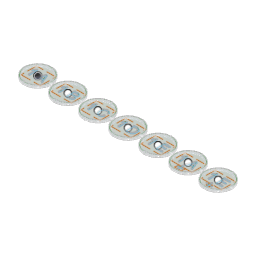
_Marker Chip 1A.5286f14f-15ed-4947-bf56-e78f0308ec14 (Autodesk Fusion 360 design; units mm, degrees)
Autodesk Fusion 360 part; units mm, degrees
sketch "Sketch4" plane through (0, 0, 0) normal (0, 0, 1) x (1, 0, 0)
  circle A0 centre (0, 0) radius 15.875
  circle A1 centre (0, 0) radius 14.2875
  line L0 (-10.8249, -8.5014) -> (11.483, -8.5014) construction
  line L1 (11.483, -8.5014) -> (11.483, 9.3249) construction
  line L2 (11.483, 9.3249) -> (-10.8249, 9.3249) construction
  line L3 (-10.8249, 9.3249) -> (-10.8249, -8.5014) construction
  circle A2 centre (34.925, 0) radius 14.2875
  circle A3 centre (34.925, 0) radius 15.875
  circle A4 centre (69.85, 0) radius 14.2875
  circle A5 centre (69.85, 0) radius 15.875
  circle A6 centre (104.775, 0) radius 14.2875
  circle A7 centre (104.775, 0) radius 15.875
  circle A8 centre (139.7, 0) radius 14.2875
  circle A9 centre (139.7, 0) radius 15.875
  circle A10 centre (174.625, 0) radius 14.2875
  circle A11 centre (174.625, 0) radius 15.875
  circle A12 centre (209.55, 0) radius 14.2875
  circle A13 centre (209.55, 0) radius 15.875
  line L4 (23.5786, -7.8769) -> (46.845, -7.8769) construction
  line L5 (46.845, -7.8769) -> (46.845, 8.6829) construction
  line L6 (46.845, 8.6829) -> (23.5786, 8.6829) construction
  line L7 (23.5786, 8.6829) -> (23.5786, -7.8769) construction
  line L8 (59.2416, -9.118) -> (81.1009, -8.8062) construction
  line L9 (81.1009, -8.8062) -> (80.8387, 9.5833) construction
  line L10 (80.8387, 9.5833) -> (58.9793, 9.2715) construction
  line L11 (58.9793, 9.2715) -> (59.2416, -9.118) construction
  line L12 (93.5032, -8.1758) -> (116.492, -8.1758) construction
  line L13 (116.492, -8.1758) -> (116.492, 8.7795) construction
  line L14 (116.492, 8.7795) -> (93.5032, 8.7795) construction
  line L15 (93.5032, 8.7795) -> (93.5032, -8.1758) construction
  line L16 (128.3241, -8.4065) -> (151.2526, -8.4065) construction
  line L17 (151.2526, -8.4065) -> (151.2526, 8.6441) construction
  line L18 (151.2526, 8.6441) -> (128.3241, 8.6441) construction
  line L19 (128.3241, 8.6441) -> (128.3241, -8.4065) construction
  line L20 (162.9563, -7.693) -> (186.6646, -7.693) construction
  line L21 (186.6646, -7.693) -> (186.6646, 8.2447) construction
  line L22 (186.6646, 8.2447) -> (162.9563, 8.2447) construction
  line L23 (162.9563, 8.2447) -> (162.9563, -7.693) construction
  line L24 (171.4525, -12.3389) -> (179.0736, -12.3282) construction
  line L25 (179.0736, -12.3282) -> (179.0675, -7.9811) construction
  line L26 (179.0675, -7.9811) -> (171.4464, -7.9918) construction
  line L27 (171.4464, -7.9918) -> (171.4525, -12.3389) construction
  line L28 (197.9424, -8.0388) -> (221.3614, -8.0388) construction
  line L29 (221.3614, -8.0388) -> (221.3614, 8.3305) construction
  line L30 (221.3614, 8.3305) -> (197.9424, 8.3305) construction
  line L31 (197.9424, 8.3305) -> (197.9424, -8.0388) construction
  line L32 (207.8072, -11.8902) -> (211.3487, -11.8813) construction
  line L33 (211.3487, -11.8813) -> (211.341, -8.8147) construction
  line L34 (211.341, -8.8147) -> (207.7995, -8.8235) construction
  line L35 (207.7995, -8.8235) -> (207.8072, -11.8902) construction
  point P0 (34.925, 0)
  point P1 (69.85, 0)
  point P2 (104.775, 0)
  point P3 (139.7, 0)
  point P4 (174.625, 0)
  point P5 (209.55, 0)
  dimension "d14" = 31.75
  dimension "d19" = 28.575
  dimension "d20" = 10.0076
  dimension "d23" = 34.925
  dimension "d24" = 0
  dimension "d25" = 10.0076
  dimension "d26" = 10.0076
  dimension "d27" = 10.0076
  dimension "d28" = 10.0076
  dimension "d29" = 10.0076
  dimension "d30" = 10.0076
  dimension "d31" = 10.0076
  dimension "d32" = 10.0076
  text T0 "1 A" font "Arial" height 10.0076 align centre middle in box 22.3079 x 17.8263 at (-10.8249, -8.5014) x (1, 0) y (0, 1) spacing 1 kerned
  text T1 "1 B" font "Arial" height 10.0076 align centre middle in box 23.2664 x 16.5598 at (23.5786, -7.8769) x (1, 0) y (0, 1) spacing 1 kerned
  text T2 "1 C" font "Arial" height 10.0076 align centre middle in box 21.8615 x 18.3914 at (59.2416, -9.118) x (0.999898, 0.014262) y (-0.014262, 0.999898) spacing 1 kerned
  text T3 "1 D" font "Arial" height 10.0076 align centre middle in box 22.9888 x 16.9553 at (93.5032, -8.1758) x (1, 0) y (0, 1) spacing 1 kerned
  text T4 "1 E" font "Arial" height 10.0076 align centre middle in box 22.9286 x 17.0506 at (128.3241, -8.4065) x (1, 0) y (0, 1) spacing 1 kerned
  text T5 "1 A" font "Arial" height 10.0076 align centre middle in box 23.7082 x 15.9377 at (162.9563, -7.693) x (1, 0) y (0, 1) spacing 1 kerned
  text T6 "+" font "Arial" height 10.0076 align centre middle in box 7.6211 x 4.3471 at (171.4525, -12.3389) x (0.999999, 0.001408) y (-0.001408, 0.999999) spacing 1 kerned
  text T7 "1 E" font "Arial" height 10.0076 align centre middle in box 23.419 x 16.3693 at (197.9424, -8.0388) x (1, 0) y (0, 1) spacing 1 kerned
  text T8 "+" font "Arial" height 10.0076 align centre middle in box 3.5415 x 3.0666 at (207.8072, -11.8902) x (0.999997, 0.002489) y (-0.002489, 0.999997) spacing 1 kerned
  constraint coincident A0.centre A1.centre
  constraint coincident A1
  constraint coincident A2
  constraint coincident A4
  constraint coincident A6
  constraint coincident A8
  constraint coincident A10
  constraint coincident A12
  measures "d14" diameter of A0
  measures "d19" diameter of A1
extrude "Extrude1" add sketch "Sketch4" sketch "Sketch4" against normal blind 1 contours A0 | A1 | A2 | A3 | A4 | A5 | A6 | A7 | A8 | A9 | A10 | A11 | A12 | A13 of sketch 2 text T0 T7 makes body 1 at (138.5225, 5.159, 0) makes body 2 at (4.6653, 4.9259, 0) makes body 3 at (105.1704, 5.0411, 0) makes body 4 at (173.4475, 5.159, 0) makes body 5 at (38.4594, -5.6969, 0) makes body 6 at (73.9314, 4.2551, 0) makes body 7 at (208.3725, 5.159, 0) in component "Bases"
extrude "Extrude1'" add sketch "Sketch4" sketch "Sketch4" along normal blind 1 separate body of sketch 2 text T0 T2 T3 T4 T5 T7 T8 T6 T1 makes body 8 at (130.7855, -12.4434, 0) makes body 9 at (15.2335, -1.4985, 0) makes body 10 at (162.4388, -9.263, 0) makes body 11 at (29.1294, 1.3587, 0) makes body 12 at (175.0688, -11.744, 0) makes body 13 at (203.573, 1.1015, 0) makes body 14 at (168.7315, 1.2316, 0) makes body 15 at (133.7094, 1.0745, 0) makes body 16 at (98.5296, 1.2576, 0) makes body 17 at (63.4635, 1.0947, 0) makes body 18 at (-5.7499, 1.3675, 0) makes body 19 at (7.2909, 0.1137, 0) makes body 20 at (71.5234, 0.9284, 0) makes body 21 at (106.9102, -0.9724, 0) makes body 22 at (142.1173, -0.02, 0) makes body 23 at (181.7723, -0.0222, 0) makes body 24 at (211.9809, 0.007, 0) makes body 25 at (209.7733, -12.6661, 0) makes body 26 at (37.4555, 0.2756, 0) makes body 27 at (120.0085, -1.4985, 0) makes body 28 at (50.1585, -1.4985, 0) makes body 29 at (85.1367, -0.7887, 0) makes body 30 at (200.6355, -12.4434, 0) in component "Chips"
sketch "Sketch3" plane through (0, 0, 0) normal (0, 0, 1) x (1, 0, 0)
  circle A0 centre (0, 0) radius 15.875
  dimension "d13" = 31.75
  constraint coincident A0.centre origin
  measures "d13" diameter of A0
component "Bases" placed x (1, 0, 0) y (0, 1, 0) z (0, 0, 1) at (0, 0, 0)
component "Chips" placed x (1, 0, 0) y (0, 1, 0) z (0, 0, 1) at (0, 0, 0)
equation "d14 = Dia"
equation "Dia = 1.25 in"
equation "Ring = 1.125 in"
equation "Thick = 1 mm"
equation "Base = 1 mm"
equation "d19 = Ring"
equation "d23 = Dia + 0.125 in"
equation "d35 = -Base"
equation "d37 = Thick"
